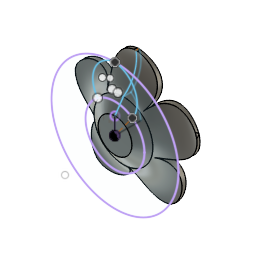
flower (Autodesk Fusion 360 design; units mm, degrees)
part number: 2026-02-27-18-31-19-793
Autodesk Fusion 360 part; units mm, degrees
sketch "Sketch7" plane through (0, 0, 0) normal (1, 0, 0) x (0, 1, 0)
  line L0 (0, 0) -> (0, 20.108)
  line L1 (0, 20.108) -> (10.0186, 35)
  line L2 (0, 0) -> (30.8415, 0)
  line L3 (10.0186, 35) -> (19, 35)
  arc A0 (19, 35) -> (28.258, 75.4678) centre (-5.8416, 61.976) ccw
  arc A1 (10.0186, 35) -> (25, 75) centre (-15.0467, 67.1934) ccw
  line L4 (25, 75) -> (28.258, 75.4678) construction
  line L5 (25, 75) -> (28.258, 75.4678)
  arc A2 (30.8415, 0) -> (19, 35) centre (-59.3948, -11.0264) ccw
  constraint coincident L0.start L2.start
  constraint vertical L0
  constraint perpendicular L0 L2
  constraint horizontal L3
  constraint coincident L3 L1.end
revolve "Revolve3" add sketch "Sketch7" angle 360 about axis through (0, 0, 0) along (0, 1, 0) contours L0 L1 L2 L3 A2 makes body 1
revolve "Revolve4" add sketch "Sketch7" angle 360 about axis through (0, 0, 0) along (0, 1, 0) contours L3 A0 A1 L5 bodies 1
sketch "Sketch8" plane through (0, 0, 0) normal (0, 1, 0) x (1, 0, 0)
  circle A0 centre (0, 0) radius 75.4678
  circle A1 centre (0, 0) radius 35
  circle A2 centre (0, 0) radius 75.4678
  circle A3 centre (0, 0) radius 35
  line L0 (0, 0) -> (20.6084, -28.2894) construction
  arc A4 (-0.0022, -75.4678) -> (20.6084, -28.2894) centre (-3.4969, -45.8498) ccw
  line L1 (0, 0) -> (0, -20.108)
  arc A5 (-20.6084, -28.2894) -> (0.0022, -75.4678) centre (3.4969, -45.8498) ccw
  constraint coincident A0.centre A1.centre
  constraint coincident A3 L0.end
  constraint tangent L0 A4
  constraint coincident A2 A4.start
  constraint symmetric L0.end L1 A5.start
  constraint symmetric A4.start L1 A5.end
  constraint symmetric A4 L1 A5
extrude "Extrude3" cut sketch "Sketch8" along normal blind 40 contours A1 A3 A4 A5 keep common part bodies 1
pattern_circular "C-Pattern1" count 5 over 360 about axis through (0, 0, 0) along (0, 1, 0) of bodies 1 makes body 2 at (36.9422, 12.3519, 1.1794) makes body 3 at (12.5374, 12.3519, -34.7696) makes body 4 at (-29.1936, 12.3519, -22.6682) makes body 5 at (-30.5801, 12.3519, 20.7599)
revolve "Revolve5" add sketch "Sketch7" angle 360 about axis through (0, 0, 0) along (0, 1, 0) contours L0 L1 L2 L3 A2 bodies 1 2 3 4 5
sketch "Sketch9" plane through (0, 0, 0) normal (0, 1, 0) x (1, 0, 0)
  circle A0 centre (0, 0) radius 3
  dimension "d16" = 6
  constraint coincident A0.centre origin
  measures "d16" diameter of A0
extrude "Extrude4" [suppressed]
